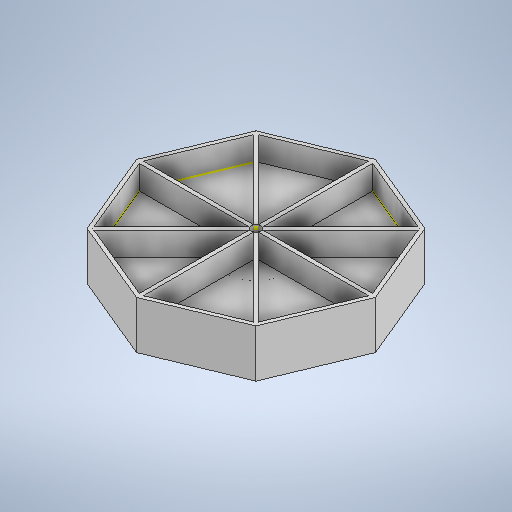
# Autodesk Inventor part: Część1
Saved by Autodesk Inventor 2025 (Build 290162000, 162)
## iProperties
Created: 2024-12-30
Part Number: Część1
Material: Ogólny
Document SubType Name: Modeling
Designer: Laptop
Density: 1 g/cm^3
Appearance: Domyślna
Author: Laptop
Autodesk Inventor part; units mm, degrees
ref_plane "YZ Plane" through (0, 0, 0) normal (1, 0, 0) x (0, 1, 0)
ref_plane "XZ Plane" through (0, 0, 0) normal (0, 1, 0) x (-1, 0, 0)
ref_plane "XY Plane" through (0, 0, 0) normal (0, 0, 1) x (1, 0, 0)
sketch "Szkic3" plane through (0, 0, 0) normal (0, 1, 0) x (-1, 0, 0)
  line L0 (0, 150) -> (106.066, 106.066)
  line L1 (106.066, 106.066) -> (150, 0)
  line L2 (150, 0) -> (106.066, -106.066)
  line L3 (106.066, -106.066) -> (0, -150)
  line L4 (0, -150) -> (-106.066, -106.066)
  line L5 (-106.066, -106.066) -> (-150, 0)
  line L6 (-150, 0) -> (-106.066, 106.066)
  line L7 (-106.066, 106.066) -> (0, 150)
  point P0 (0, 0)
  point P1 (0, 0)
  dimension "d2" = 300
  constraints: 16 end point, 1 coincident, 17 other
  measures "d2" distance of L0.start L3.end
extrude "Wyciągnięcie proste2" add sketch "Szkic3" along normal blind 50
sketch "Szkic4" plane through (0, 50, 0) normal (0, 1, 0) x (1, 0, 0)
  point P0 (0, 0)
sketch "Szkic5" plane through (0, 50, 0) normal (0, 1, 0) x (1, 0, 0)
  line L0 (0, 145) -> (102.5305, 102.5305)
  line L1 (102.5305, 102.5305) -> (145, 0)
  line L2 (145, 0) -> (102.5305, -102.5305)
  line L3 (102.5305, -102.5305) -> (0, -145)
  line L4 (0, -145) -> (-102.5305, -102.5305)
  line L5 (-102.5305, -102.5305) -> (-145, 0)
  line L6 (-145, 0) -> (-102.5305, 102.5305)
  line L7 (-102.5305, 102.5305) -> (0, 145)
  point P0 (0, 0)
  point P1 (0, 0)
  dimension "d5" = 290
  constraints: 16 end point, 1 coincident, 17 other
  measures "d5" distance of L3.end L0.start
extrude "Wyciągnięcie proste3" cut sketch "Szkic5" against normal blind 30
sketch "Szkic6" plane through (0, 20, 0) normal (0, 1, 0) x (1, 0, 0)
  line L0 (-102.5305, -102.5305) -> (-145, 0) projected
  line L1 (0, 145) -> (102.5305, 102.5305) projected
  line L2 (-145, 0) -> (-102.5305, 102.5305) projected
  line L3 (145, 0) -> (102.5305, -102.5305) projected
  line L4 (0, -145) -> (-102.5305, -102.5305) projected
sketch "Szkic7" plane through (0, 20, 0) normal (0, 1, 0) x (1, 0, 0)
  line L0 (-145, 0) -> (-102.5305, 102.5305) projected
  line L1 (-145, 2.5) -> (145, 2.5)
  line L2 (145, 2.5) -> (145, -2.5)
  line L3 (145, -2.5) -> (-145, -2.5)
  line L4 (-145, -2.5) -> (-145, 2.5)
  line L5 (-145, 2.5) -> (145, -2.5) construction
  line L6 (145, 2.5) -> (-145, -2.5) construction
  line L7 (-2.5, 145) -> (-2.5, -145)
  line L8 (-2.5, -145) -> (2.5, -145)
  line L9 (2.5, -145) -> (2.5, 145)
  line L10 (2.5, 145) -> (-2.5, 145)
  line L11 (-2.5, 145) -> (2.5, -145) construction
  line L12 (-2.5, -145) -> (2.5, 145) construction
  line L13 (100.7627, -104.2983) -> (-104.2983, 100.7627)
  line L14 (-104.2983, 100.7627) -> (-100.7627, 104.2983)
  line L15 (-100.7627, 104.2983) -> (104.2983, -100.7627)
  line L16 (104.2983, -100.7627) -> (100.7627, -104.2983)
  line L17 (100.7627, -104.2983) -> (-100.7627, 104.2983) construction
  line L18 (-104.2983, 100.7627) -> (104.2983, -100.7627) construction
  line L19 (100.7322, 104.2678) -> (-104.2678, -100.7322)
  line L20 (-104.2678, -100.7322) -> (-100.7322, -104.2678)
  line L21 (-100.7322, -104.2678) -> (104.2678, 100.7322)
  line L22 (104.2678, 100.7322) -> (100.7322, 104.2678)
  line L23 (100.7322, 104.2678) -> (-100.7322, -104.2678) construction
  line L24 (-104.2678, -100.7322) -> (104.2678, 100.7322) construction
  point P0 (0, 0)
  point P1 (-6.0355, 2.5)
  point P2 (-6.0355, -2.5)
  point P3 (-2.5, -6.0355)
  point P4 (2.5, -6.0355)
  point P5 (6.0355, -2.5)
  point P6 (6.0355, 2.5)
  point P7 (2.5, 6.0355)
  point P8 (-2.5, 6.0355)
  dimension "d11" = 5
  dimension "d12" = 5
  dimension "d13" = 5
  dimension "d14" = 5
  constraints: 48 end point, 9 parallel, 8 midpoint, 4 perpendicular, 1 horizontal
  measures "d11" distance of L1.end L2.end
  measures "d12" distance of L8.end L7.end
  measures "d13" distance of L13.end L14.end
  measures "d14" distance of L20.end L19.end
extrude "Wyciągnięcie proste4" add sketch "Szkic7" along normal blind 30 contours L4 L1 L0 | L0 L1 L13 L19 L3 L4 | L13 L14 L0 | L0 L14 L15 L7 L1 L13 | L1 L7 L19 L13 | L19 L13 L7 L3 | L3 L7 L21 L20 L19 | L7 L15 L19 L1 | L1 L19 L7 | L19 L7 L13 | L7 L13 L3 | L3 L13 L21 L7 | L19 L15 L1 | L1 L15 L9 L21 L3 L13 L7 L19 | L7 L10 L9 L19 L15 | L3 L21 L13 | L21 L13 L9 L8 L7 | L15 L19 L9 L1 | L1 L9 L15 | L21 L9 L3 | L3 L9 L13 L21 | L9 L19 L22 L21 L1 | L1 L21 L15 L9 | L15 L21 L9 | L9 L21 L15 L3 | L3 L15 L16 L13 L9 | L1 L2 L3 L15 L21
sketch "Szkic8" plane through (0, 50, 0) normal (0, 1, 0) x (1, 0, 0)
  circle A0 centre (0, 0) radius 6
  dimension "d17" = 12
  constraints: 1 centre point, 1 coincident
  measures "d17" diameter of A0
extrude "Wyciągnięcie proste5" cut sketch "Szkic8" against normal blind 12
sketch "Szkic9" plane through (0, 0, 0) normal (0, -1, 0) x (1, 0, 0)
  circle A0 centre (0, 0) radius 37.5
  dimension "d20" = 75
  constraints: 1 centre point, 1 coincident
  measures "d20" diameter of A0
extrude "Wyciągnięcie proste6" cut sketch "Szkic9" against normal blind 19
sketch "Szkic10" plane through (0, 0, 0) normal (0, -1, 0) x (1, 0, 0)
  point P0 (0, 0)
sketch "Szkic11" plane through (0, 0, 0) normal (0, -1, 0) x (1, 0, 0)
  circle A0 centre (0, 0) radius 37.5 projected
  line L0 (106.066, 106.066) -> (150, 0) projected
  line L1 (0, 150) -> (106.066, 106.066) projected
  line L2 (-106.066, 106.066) -> (0, 150) projected
  line L3 (-150, 0) -> (-106.066, 106.066) projected
  line L4 (-106.066, -106.066) -> (-150, 0) projected
  line L5 (0, -150) -> (-106.066, -106.066) projected
  line L6 (106.066, -106.066) -> (0, -150) projected
  line L7 (150, 0) -> (106.066, -106.066) projected
  circle A1 centre (0, 0) radius 37.5 projected
  line L8 (106.066, 106.066) -> (150, 0) projected
  line L9 (0, 150) -> (106.066, 106.066) projected
  line L10 (-106.066, 106.066) -> (0, 150) projected
  line L11 (-150, 0) -> (-106.066, 106.066) projected
  line L12 (-106.066, -106.066) -> (-150, 0) projected
  line L13 (0, -150) -> (-106.066, -106.066) projected
  line L14 (106.066, -106.066) -> (0, -150) projected
  line L15 (150, 0) -> (106.066, -106.066) projected
extrude "Wyciągnięcie proste7" add sketch "Szkic11" along normal blind 10
equation "\"d18\" = d17"
